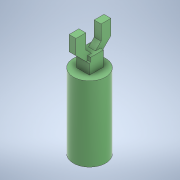
# Autodesk Inventor part: czesc5
Saved by Autodesk Inventor 2022 (Build 260153000, 153)
## iProperties
Created: 2022-06-07
Part Number: czesc5
Material: Ogólny
Document SubType Name: Sheet Metal
Designer: admin
Density: 1 g/cm^3
Sheet Metal Rule: Domyślny_mm
Appearance: Domyślna
Author: admin
Autodesk Inventor part; units mm, degrees
ref_plane "YZ Plane" through (0, 0, 0) normal (1, 0, 0) x (0, 1, 0)
ref_plane "XZ Plane" through (0, 0, 0) normal (0, 1, 0) x (-1, 0, 0)
sketch "Szkic1" plane through (0, 0, 0) normal (0, 1, 0) x (-1, 0, 0)
  circle A0 centre (0, 0) radius 12.5
  circle A1 centre (0, 0) radius 32.5
  dimension "d0" = 25
  dimension "d1" = 65
  constraints: 2 centre point, 2 coincident
  measures "d0" diameter of A0
  measures "d1" diameter of A1
extrude "Wyciągnięcie proste1" add sketch "Szkic1" along normal blind 150 contours A0 | A1
sketch "Szkic2" plane through (0, 0, 0) normal (0, -1, 0) x (1, 0, 0)
  point P0 (0, 0)
extrude "Wyciągnięcie proste2" cut sketch "Szkic1" along normal blind 100 contours A0
sketch "Szkic3" plane through (0, 150, 0) normal (0, 1, 0) x (1, 0, 0)
  line L0 (13, -13) -> (-13, -13)
  line L1 (-13, -13) -> (-13, 13)
  line L2 (-13, 13) -> (13, 13)
  line L3 (13, 13) -> (13, -13)
  line L4 (13, -13) -> (-13, 13) construction
  line L5 (-13, -13) -> (13, 13) construction
  point P0 (0, 0)
  dimension "d6" = 26
  dimension "d7" = 26
  constraints: 12 end point, 2 midpoint, 2 parallel, 1 horizontal, 1 perpendicular
  measures "d6" distance of L1.end L2.end
  measures "d7" distance between parallel lines of L2 L0
extrude "Wyciągnięcie proste3" add sketch "Szkic3" along normal blind 30
chamfer "Faza1" distance 10 angle 45 2 edges at (0, 180, -13) (0, 180, 13)
sketch "Szkic4" plane through (-13, 180, 3) normal (0, 0.7071, 0.7071) x (1, 0, 0)
  line L0 (26, 0) -> (0, 0) projected
  line L1 (6, -14) -> (20, -14)
  line L2 (20, -14) -> (20, 0)
  line L3 (20, 0) -> (6, 0)
  line L4 (6, 0) -> (6, -14)
  line L5 (6, -14) -> (20, 0) construction
  line L6 (20, -14) -> (6, 0) construction
  line L7 (0, 0) -> (0, -14.1421) projected
  point P0 (13, -125.1579)
  point P1 (13, -7)
  dimension "d13" = 14
  dimension "d14" = 14
  dimension "d15" = 6
  constraints: 12 end point, 2 midpoint, 2 parallel, 1 horizontal, 1 perpendicular, 1 point on line
  measures "d13" distance of L1.end L2.end
  measures "d14" distance between parallel lines of L4 L2
  measures "d15" distance between parallel lines of L7 L4
extrude "Wyciągnięcie proste4" add sketch "Szkic4" along normal blind 30
chamfer "Faza2" distance 14 angle 45 1 edges at (0, 201.2132, 24.2132)
sketch "Szkic5" plane through (-7, 191.3137, 34.1127) normal (0, 1, 0) x (1, 0, 0)
  line L0 (0, 31.1127) -> (0, 19.799) projected
  line L1 (14, 0) -> (0, 0)
  line L2 (0, 0) -> (0, 19.799)
  line L3 (0, 19.799) -> (14, 19.799)
  line L4 (14, 19.799) -> (14, 0)
  point P0 (7, 34.1127)
  dimension "d21" = 14
  dimension "d22" = 19.799
  constraints: 8 end point, 2 parallel, 1 horizontal, 1 perpendicular
  measures "d21" distance between parallel lines of L4 L0
  measures "d22" distance between parallel lines of L3 L1
extrude "Wyciągnięcie proste5" add sketch "Szkic5" along normal blind 30
ref_plane "Płaszczyzna konstrukcyjna1" through (-13, 150, -1) normal (0, 0, 1) x (1, 0, 0)
mirror "Odbij1" about plane through (-13, 150, -1) normal (0, 0, 1) of "Wyciągnięcie proste5", "Wyciągnięcie proste4", "Wyciągnięcie proste3"
equation "\"PromieńGięcia\" = Grubość"
equation "\"SzerokośćGięciaPodcięcia\" = Grubość"
equation "\"GłębokośćGięciaPodcięcia\" = 0.5 * Grubość"
equation "\"RozmiarPodcięciaNarożnika\" = 4 * Grubość"
equation "\"MinimalnaPozostałość\" = 2 * Grubość"
equation "\"PromieńPrzejścia\" = PromieńGięcia"
equation "\"Rozmiar_promienia_Jacobiego\" = PromieńGięcia"
equation "\"Wielk_odstępu\" = Grubość"
equation "\"Grubość\" = 0.5"
